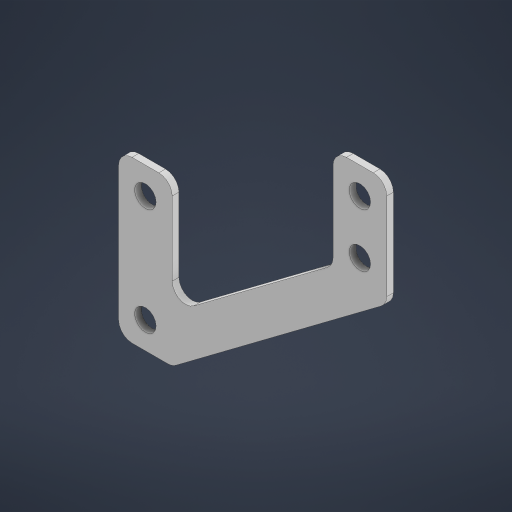
# Autodesk Inventor part: funnelPoly
Saved by Autodesk Inventor 2023.4 (Build 274418000, 418)
## iProperties
Created: 2024-03-08
Part Number: funnelPoly
Material: Generic
Document SubType Name: Modeling
Designer: Meer
Density: 1 g/cm^3
Appearance: Default
Author: Meer
Autodesk Inventor part; units mm, degrees
ref_plane "YZ Plane" through (0, 0, 0) normal (1, 0, 0) x (0, 1, 0)
ref_plane "XZ Plane" through (0, 0, 0) normal (0, 1, 0) x (-1, 0, 0)
ref_plane "XY Plane" through (0, 0, 0) normal (0, 0, 1) x (1, 0, 0)
sketch "Sketch1" plane through (0, 0, 0) normal (0, 0, 1) x (1, 0, 0)
  line L0 (0, 0) -> (50.8, 0)
  line L1 (50.8, 0) -> (50.8, 50.8)
  line L2 (50.8, 50.8) -> (0, 50.8)
  line L3 (0, 50.8) -> (0, 0)
  circle A0 centre (50.8, 50.8) radius 2.54
  line L4 (50.8, 50.8) -> (50.8, 38.1)
  circle A1 centre (50.8, 38.1) radius 2.54
  line L5 (50.8, 50.8) -> (50.8, 57.15)
  line L6 (50.8, 57.15) -> (57.15, 57.15)
  line L7 (57.15, 57.15) -> (57.15, 50.8)
  line L8 (57.15, 50.8) -> (57.15, 0)
  line L9 (50.8, 57.15) -> (0, 57.15)
  line L10 (50.8, 57.15) -> (44.45, 57.15)
  line L11 (44.45, 57.15) -> (44.45, 31.75)
  line L12 (44.45, 31.75) -> (57.15, 31.75)
  circle A2 centre (0, 0) radius 2.54
  line L13 (0, 0) -> (0, -6.35)
  line L14 (0, -6.35) -> (6.35, -6.35)
  line L15 (6.35, -6.35) -> (6.35, 0)
  line L16 (0, 0) -> (-6.35, 0)
  line L17 (-6.35, 0) -> (-6.35, -6.35)
  line L18 (-6.35, -6.35) -> (0, -6.35)
  line L19 (0, 0) -> (0, 25.4)
  circle A3 centre (0, 25.4) radius 2.54
  line L20 (-6.35, 0) -> (-6.35, 31.75)
  line L21 (-6.35, 31.75) -> (6.35, 31.75)
  line L22 (6.35, 31.75) -> (6.35, 0)
  line L23 (6.35, -6.35) -> (57.15, 31.75)
  line L24 (44.45, 31.75) -> (44.45, 22.225)
  line L25 (6.35, -6.35) -> (6.35, 3.175)
  line L26 (50.8, 38.1) -> (0, 0)
  point P0 (44.45, 33.3375)
  point P1 (6.35, 4.7625)
  dimension "d1" = 50.8
  dimension "d2" = 50.8
  dimension "d3" = 5.08
  dimension "d4" = 12.7
  dimension "d5" = 5.08
  dimension "d6" = 6.35
  dimension "d7" = 6.35
  dimension "d8" = 6.35
  dimension "d9" = 50.8
  dimension "d10" = 50.8
  dimension "d11" = 6.35
  dimension "d12" = 25.4
  dimension "d13" = 5.08
  dimension "d14" = 6.35
  dimension "d15" = 6.35
  dimension "d16" = 6.35
  dimension "d17" = 25.4
  dimension "d18" = 5.08
  dimension "d19" = 9.525
  constraints: 54 end point, 12 perpendicular, 10 point on line, 4 centre point, 4 coincident, 3 equal length, 2 horizontal, 1 midpoint, 1 vertical
  measures "d1" distance of L2.end L1.end
  measures "d2" distance of L1.end L0.end
  measures "d3" diameter of A0
  measures "d4" distance of L4.start L4.end
  measures "d5" diameter of A1
  measures "d6" distance of L4.start L5.end
  measures "d7" distance of L5.end L6.end
  measures "d8" distance of L6.end L7.end
  measures "d9" distance of L5.end L9.end
  measures "d10" distance of L7.end L8.end
  measures "d11" distance of L5.end L10.end
  measures "d12" distance of L10.end L11.end
  measures "d13" diameter of A2
  measures "d14" distance of L13.start L13.end
  measures "d15" distance of L13.end L14.end
  measures "d16" distance of L13.start L16.end
  measures "d17" distance of L13.start L19.end
  measures "d18" diameter of A3
  measures "d19" distance of L14.end L25.end
extrude "Extrusion1" add sketch "Sketch1" along normal blind 1.5875 contours A2 L26 L22 L0 | L0 L15 L14 L13 A2 | A2 L16 L20 L21 L3 A3 | L3 A3 L21 L22 L26 A2 | L13 L18 L17 L16 A2 | L22 L26 L11 L24 L23 L0 | L0 L23 L15 | L26 A1 L1 L12 L11 | L11 L2 A0 L1 A1 L26 | L24 L12 L1 L23 | L11 L9 L5 A0 L2 | L1 L12 L23 | L1 A1 A0 L5 L6 L7 L8 L12
fillet "Fillet1" radius 3.175 9 edges at (-6.35, 31.75, 0.7937) (6.35, 31.75, 0.7937) (-6.35, -6.35, 0.7937) (6.35, -6.35, 0.7937) (6.35, 4.7625, 0.7937) (44.45, 33.3375, 0.7937) (44.45, 57.15, 0.7937) (57.15, 57.15, 0.7937) (57.15, 31.75, 0.7937)
body "Solid1"
